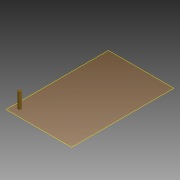
# Autodesk Inventor part: nanopc_t4_spacer_long
Saved by Autodesk Inventor 2013 SP2 (Build 170200200, 200)
## iProperties
Created: 2018-09-03
Part Number: nanopc_t4_spacer_long
Material: Brass, Soft Yellow
Document SubType Name: Modeling
Designer: alex
Density: 8.47 g/cm^3
Author: alex
Autodesk Inventor part; units mm, degrees
ref_plane "YZ Plane" through (0, 0, 0) normal (1, 0, 0) x (0, 1, 0)
ref_plane "XZ Plane" through (0, 0, 0) normal (0, 1, 0) x (-1, 0, 0)
ref_plane "XY Plane" through (0, 0, 0) normal (0, 0, 1) x (1, 0, 0)
ref_plane "Work Plane1" through (0, 0, 0) normal (0, 0, 1) x (1, 0, 0)
sketch "Sketch1" plane through (0, 0, 0) normal (0, 0, 1) x (1, 0, 0)
  circle A0 centre (-28.8, -46.8) radius 1.6 projected
  line L0 (-27.8762, -45.2) -> (-26.9525, -46.8)
  line L1 (-26.9525, -46.8) -> (-27.8762, -48.4)
  line L2 (-27.8762, -48.4) -> (-29.7238, -48.4)
  line L3 (-29.7238, -48.4) -> (-30.6475, -46.8)
  line L4 (-30.6475, -46.8) -> (-29.7238, -45.2)
  line L5 (-29.7238, -45.2) -> (-27.8762, -45.2)
  point P0 (0, 0)
  point P1 (-28.8, -45.2)
  constraints: 12 end point, 1 coincident, 1 midpoint, 1 vertical alignment, 14 other
extrude "Extrusion1" add sketch "Sketch1" along normal blind 16.5
sketch "Sketch2" plane through (0, 0, 0) normal (0, 0, -1) x (-1, 0, 0)
  circle A0 centre (28.8, -46.8) radius 1.5
  point P0 (0, 0)
  dimension "d2" = 3
  constraints: 1 centre point
  measures "d2" diameter of A0
extrude "Extrusion2" add sketch "Sketch2" along normal blind 6
body "Solid1"
